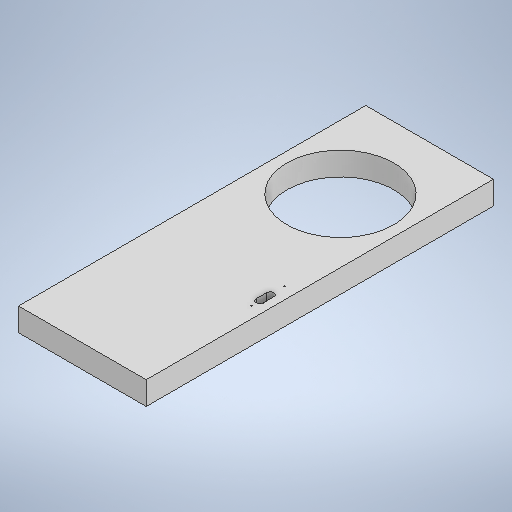
# Autodesk Inventor part: Schutz
Saved by Autodesk Inventor 2025.1 (Build 291241000, 241)
## iProperties
Created: 2024-08-07
Part Number: Schutz
Material: Generic
Document SubType Name: Modeling
Designer: ffogue
Density: 1 g/cm^3
Appearance: Default
Author: ffogue
Autodesk Inventor part; units mm, degrees
ref_plane "YZ Plane" through (0, 0, 0) normal (1, 0, 0) x (0, 1, 0)
ref_plane "XZ Plane" through (0, 0, 0) normal (0, 1, 0) x (-1, 0, 0)
ref_plane "XY Plane" through (0, 0, 0) normal (0, 0, 1) x (1, 0, 0)
sketch "Sketch6" plane through (0, 0, 0) normal (0, 0, 1) x (1, 0, 0)
  line L0 (0, 0) -> (716, 0)
  line L1 (716, 0) -> (716, 1947)
  line L2 (716, 1947) -> (0, 1947)
  line L3 (0, 1947) -> (0, 0)
  dimension "d0" = 716
  dimension "d1" = 1947
  constraints: 8 end point, 2 parallel, 1 horizontal, 1 perpendicular
  measures "d0" distance between parallel lines of L1 L3
  measures "d1" distance between parallel lines of L0 L2
extrude "Extrusion1" add sketch "Sketch6" along normal mid plane 130
sketch "Sketch7" plane through (0, 0, 65) normal (0, 0, 1) x (1, 0, 0)
  circle A0 centre (358, 1447) radius 300
  line L0 (716, 1947) -> (0, 1947) projected
  point P0 (0, 0)
  point P1 (358, 1947)
  dimension "d4" = 600
  dimension "d5" = 500
  constraints: 1 centre point, 1 midpoint, 1 vertical alignment
  measures "d4" diameter of A0
  measures "d5" distance from line of L0 A0.centre
extrude "Extrusion2" cut sketch "Sketch7" against normal up to surface (130 mm away)
sketch "Sketch9" plane through (0, 0, 65) normal (0, 0, 1) x (1, 0, 0)
  line L0 (651, 761) -> (651, 701) construction
  line L1 (671, 761) -> (671, 701)
  line L2 (631, 701) -> (631, 761)
  arc A0 (671, 761) -> (631, 761) centre (651, 761) ccw
  arc A1 (631, 701) -> (671, 701) centre (651, 701) ccw
  line L3 (0, 0) -> (716, 0) projected
  line L4 (0, 1947) -> (0, 0) projected
  circle A2 centre (651, 841) radius 3.5
  circle A3 centre (651, 654) radius 3.5
  line L5 (716, 0) -> (716, 1947) projected
  point P0 (651, 731)
  point P1 (651, 681)
  point P2 (651, 781)
  dimension "d8" = 40
  dimension "d9" = 681
  dimension "d10" = 100
  dimension "d12" = 7
  dimension "d13" = 60
  dimension "d14" = 7
  dimension "d15" = 187
  dimension "d18" = 65
  constraints: 8 end point, 6 point on circle, 4 centre point, 4 tangent, 2 vertical alignment, 1 midpoint, 1 parallel, 1 vertical
  measures "d8" distance between parallel lines of L1 L2
  measures "d9" distance from line of L3 point (651, 681)
  measures "d10" distance of point (651, 681) point (651, 781)
  measures "d12" diameter of A2
  measures "d13" distance of point (651, 781) A2.centre
  measures "d14" diameter of A3
  measures "d15" distance of A2.centre A3.centre
  measures "d18" distance from line of L5 L0.start
extrude "Extrusion3" cut sketch "Sketch9" against normal up to surface (130 mm away)
equation "\"d0\" = SchuBrei"
equation "\"d1\" = SchuHoeh"
equation "\"d2\" = SchuDick"
equation "\"SchuDick\" = 130"
equation "\"SchuBrei\" = 716"
equation "\"SchuHoeh\" = 1947"
body "Solid1"
